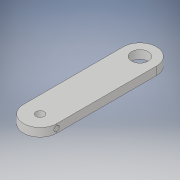
# Autodesk Inventor part: BT001_trajan20_21
Saved by Autodesk Inventor 2022.2 (Build 262287000, 287)
## iProperties
Company: HTBLA Kaindorf
RuleStatus: InUse
Created: 2022-08-07
Part Number: BT001_trajan20_21
Project: Zeichenmaschine_v2
Material: Generisch
Description: gelenk 1
Document SubType Name: Modeling
Designer: trajan20
Density: 1 g/cm^3
Appearance: Vorgabe
Mass: 7.01702 g
Surface Area: 40.4356 cm^2
Volume: 7.01702 cm^3
AfterDocNew0: iProperties-Editor_aufrufen
Author: jan
Keywords: 2021
Autodesk Inventor part; units mm, degrees
ref_plane "YZ Plane" through (0, 0, 0) normal (1, 0, 0) x (0, 1, 0)
ref_plane "XZ Plane" through (0, 0, 0) normal (0, 1, 0) x (-1, 0, 0)
ref_plane "XY Plane" through (0, 0, 0) normal (0, 0, 1) x (1, 0, 0)
sketch "Skizze3" plane through (0, 0, 0) normal (0, 0, 1) x (1, 0, 0)
  line L0 (0, 0) -> (-60, 0) construction
  line L1 (0, 10) -> (-60, 10)
  line L2 (-60, -10) -> (0, -10)
  arc A0 (0, -10) -> (0, 10) centre (0, 0) ccw
  arc A1 (-60, 10) -> (-60, -10) centre (-60, 0) ccw
  circle A2 centre (0, 0) radius 2.5
  circle A3 centre (-60, 0) radius 5
  point P0 (-30, 0)
  point P1 (-40, 0)
  dimension "d4" = 60
  dimension "d5" = 20
  dimension "d6" = 10
  dimension "d7" = 5
  dimension "d8" = 40
  constraints: 8 end point, 4 centre point, 4 point on circle, 4 tangent, 2 coincident, 1 horizontal, 1 midpoint, 1 parallel, 1 point on line
  measures "d4" distance of L0.end L0.start
  measures "d5" distance between parallel lines of L2 L1
  measures "d6" diameter of A3
  measures "d7" diameter of A2
  measures "d8" distance of L0.start point (-40, 0)
extrude "Extrusion3" add sketch "Skizze3" along normal blind 5
sketch "Skizze4" plane through (-60, 10, 0) normal (0, 1, 0) x (1, 0, 0)
  line L0 (60, 0) -> (60, -5) projected
  point P0 (60, -2.5)
  constraints: 1 midpoint
hole "Bohrung1" at (0, 10, 2.5) direction (0, -1, 0) diameter 3.242 end up to face face through (0, 0, 0) facing (0, 0, 1) round with radius 2.5 far side no thread size "M4x0.7" class "6H" standard "ISO Metric profile"
